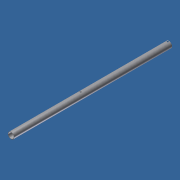
# Autodesk Inventor part: J001401
Saved by Autodesk Inventor 2012 SP2 (Build 160219200, 219)
## iProperties
Created: 2012-04-05
Material: STAINLESS STEEL, 304
Vendor: MCMASTER
Document SubType Name: Modeling
Designer: NEGRASHOVI
Density: 8 g/cm^3
Description: MCMASTER_8457K576_STAILESS STEEL TUBE 0.5 OD
Mass: 67.8444 g
Surface Area: 239.345 cm^2
Volume: 8.48054 cm^3
Part Number: J001401
Project: P-51601
RuleStatus: InUse
AfterDocSave0: file://Part Number Cleaner
LAB/DEPT: GONEN (LAB)
REQUESTING SCIENTIST: GONEN, TAMIR
SURFACE ROUGHNESS: N/A
DESIGN DEPARTMENT: HHMI: JFRC - ID&F
SPECIAL FINISH: NONE
ALTERED ITEM PART NUMBER: N/A
ALTERED ITEM VENDOR: N/A
ALTERED ITEM DESCRIPTION: N/A
Author: NEGRASHOVI
Revision Number: -
Autodesk Inventor part; units mm, degrees
ref_plane "YZ Plane" through (0, 0, 0) normal (1, 0, 0) x (0, 1, 0)
ref_plane "XZ Plane" through (0, 0, 0) normal (0, 1, 0) x (-1, 0, 0)
ref_plane "XY Plane" through (0, 0, 0) normal (0, 0, 1) x (1, 0, 0)
sketch "Sketch1" plane through (0, 0, 0) normal (0, 0, 1) x (1, 0, 0)
  circle A0 centre (0, 0) radius 6.35
  circle A1 centre (0, 0) radius 5.6388
  dimension "d0" = 12.7
  dimension "d1" = 11.2776
  constraints: 2 centre point, 2 coincident
  measures "d0" diameter of A0
  measures "d1" diameter of A1
extrude "Extrusion1" add sketch "Sketch1" along normal blind 317.5
sketch "Sketch2" plane through (0, 0, 0) normal (0, 1, 0) x (-1, 0, 0)
  line L0 (0, 0) -> (0, 382.1904) construction
  circle A0 centre (0, 2.54) radius 1.6383
  circle A1 centre (0, 177.8) radius 1.6383
  line L1 (5.6388, 0) -> (-5.6388, 0) projected
  dimension "d4" = 3.2766
  dimension "d5" = 3.2766
  dimension "d6" = 2.54
  dimension "d10" = 177.8
  constraints: 2 centre point, 2 end point, 2 point on line, 1 vertical
  measures "d4" diameter of A1
  measures "d5" diameter of A0
  measures "d6" distance of A0.centre L0.start
  measures "d10" distance from line of A1.centre L1
extrude "Extrusion2" cut sketch "Sketch2" along normal through all both and the other way through all
equation "\"d4\" = d5"
body "Solid1"
